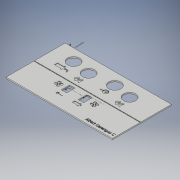
# Autodesk Inventor part: Caixa control - tapa
Saved by Autodesk Inventor 2019 (Build 230136000, 136)
## iProperties
Created: 2018-08-29
Part Number: Caixa control - tapa
Material: Genérico
Document SubType Name: Modeling
Designer: Albert Garangou Culebras
Density: 1 g/cm^3
Appearance: Valor por defecto
Author: Albert Garangou Culebras
Autodesk Inventor part; units mm, degrees
(part 1 of 2)
ref_plane "YZ Plane" through (0, 0, 0) normal (1, 0, 0) x (0, 1, 0)
ref_plane "XZ Plane" through (0, 0, 0) normal (0, 1, 0) x (-1, 0, 0)
ref_plane "XY Plane" through (0, 0, 0) normal (0, 0, 1) x (1, 0, 0)
sketch "Boceto1" plane through (0, 0, 0) normal (0, 1, 0) x (-1, 0, 0)
  line L0 (0, 0) -> (-180, 0)
  line L1 (-180, 0) -> (-180, -100)
  line L2 (-180, -100) -> (0, -100)
  line L3 (0, -100) -> (0, 0)
  dimension "d0" = 180
  dimension "d1" = 100
  constraints: 8 end point, 2 parallel, 1 horizontal, 1 perpendicular
  measures "d0" distance of L2.end L1.end
  measures "d1" distance of L1.end L0.end
extrude "base" add sketch "Boceto1" along normal blind 2
sketch "Boceto2" plane through (0, 2, 0) normal (0, 1, 0) x (1, 0, 0)
  line L0 (0, 100) -> (0, 0) projected
  line L1 (0, 0) -> (180, 0) projected
  line L2 (0, 100) -> (180, 100)
  line L3 (180, 100) -> (180, 0)
  line L4 (180, 0) -> (0, 0)
  line L5 (0, 0) -> (0, 100)
  line L6 (180, 50) -> (180, 0)
  line L7 (180, 0) -> (84.2308, 0)
  line L8 (180, 100) -> (0, 100) projected
  circle A0 centre (34.2888, 79.9235) radius 10.25
  circle A1 centre (104.2888, 79.9235) radius 10.25
  line L9 (65.4618, 35) -> (65.4618, 42)
  line L10 (65.4618, 42) -> (74.4618, 42)
  line L11 (74.4618, 42) -> (74.4618, 28)
  line L12 (74.4618, 28) -> (65.4618, 28)
  line L13 (65.4618, 28) -> (65.4618, 35)
  line L14 (94.2308, 35) -> (94.2308, 42)
  line L15 (103.2308, 42) -> (103.2308, 28)
  line L16 (103.2308, 28) -> (94.2308, 28)
  line L17 (94.2308, 28) -> (94.2308, 35)
  circle A2 centre (64.2888, 75.4263) radius 10.25
  circle A3 centre (134.2888, 74.9235) radius 10.25
  line L18 (94.2308, 42) -> (103.2308, 42)
  line L19 (94.2308, 42) -> (103.2308, 42)
  line L20 (94.2308, 42) -> (103.2308, 42)
  line L21 (103.2308, 42) -> (103.2308, 28)
  line L22 (103.2308, 28) -> (94.2308, 28)
  line L23 (94.2308, 28) -> (94.2308, 42)
  constraints: 42 end point, 8 perpendicular, 5 equal length, 4 centre point, 2 horizontal, 2 point on line, 2 vertical
sketch "Boceto5" plane through (0, 2, 0) normal (0, 1, 0) x (1, 0, 0)
  line L0 (37.6813, 63.0419) -> (37.6542, 60.4419) projected
  line L1 (37.6747, 62.4093) -> (37.6612, 61.1175)
  line L2 (41.6533, 62.4093) -> (37.6747, 62.4093)
  line L3 (41.6533, 62.4093) -> (44.1386, 62.4093) construction
  line L4 (44.1386, 62.4093) -> (44.1386, 58.5428) construction
  spline S0 degree 2 poles (41.6533, 62.4093) (44.1386, 62.4093) (44.1386, 58.5428) knots 1 1 1 2 2 2
  line L5 (41.6533, 61.1175) -> (42.896, 61.1175) construction
  line L6 (42.896, 61.1175) -> (42.896, 58.5428) construction
  spline S1 degree 2 poles (41.6533, 61.1175) (42.896, 61.1175) (42.896, 58.5428) knots 1 1 1 2 2 2
  line L7 (42.896, 58.5428) -> (44.1386, 58.5428)
  line L8 (37.6612, 61.1175) -> (41.6533, 61.1175)
  point P0 (0, 0)
  constraints: 8 end point, 3 horizontal, 2 point on line, 2 vertical, 6 other
extrude "Extrusión4" cut sketch "Boceto5" against normal blind 0.75
sketch "Boceto8" plane through (0, 2, 0) normal (0, 1, 0) x (1, 0, 0)
  spline S0 degree 4 poles (133.7635, 35.9708) (133.8407, 35.7147) (134.281, 35.6307) (134.3351, 35.9754) (134.306, 36.5115) (134.6867, 37.3994) (135.6799, 38.6611) (136.4874, 39.1799) (138.808, 38.5401) (139.0929, 36.16) knots 0 0 0 0 0 0.168165 0.246229 0.343173 0.454491 0.580711 1 1 1 1 1
  spline S1 degree 4 poles (139.0929, 36.16) (139.4262, 35.3106) (137.4111, 33.2429) (137.2359, 36.2151) (135.2011, 34.9657) knots 0 0 0 0 0 1 1 1 1 1
  spline S2 degree 3 poles (135.2011, 34.9657) (134.8312, 33.8706) (136.5984, 35.589) (138.0072, 32.8129) knots 0 0 0 0 1 1 1 1
  spline S3 degree 4 poles (134.6889, 32.599) (134.6741, 32.3205) (134.4844, 31.7908) (133.8798, 30.9164) (134.6566, 30.0496) (135.5938, 29.5497) (136.1798, 29.9491) (138.1553, 30.4347) (138.19, 32.1817) knots 0 0 0 0 0 0.26848 0.383335 0.491909 0.605906 1 1 1 1 1
  spline S4 degree 2 poles (138.19, 32.1817) (138.2278, 32.5571) (138.0072, 32.8129) knots 0 0 0 1 1 1
  spline S5 degree 3 poles (133.9221, 33.5854) (134.1222, 33.9496) (134.7297, 33.5872) (134.6889, 32.599) knots 0 0 0 0 1 1 1 1
  line L0 (134.19, 33.6433) -> (135.2195, 34.5853)
  line L1 (135.2195, 34.5853) -> (134.1584, 35.7449)
  spline S6 degree 2 poles (132.8663, 34.9339) (132.9078, 34.93) (132.9532, 34.9084) knots 0 0 0 1 1 1
  line L2 (132.9307, 34.9191) -> (132.9757, 34.8978) construction
  arc A0 (132.971, 34.8994) -> (132.935, 34.9165) centre (132.8007, 34.5869) ccw construction
  line L3 (132.9532, 34.4831) -> (134.1584, 35.7449)
  spline S7 degree 4 poles (133.9221, 33.5854) (133.6541, 32.8245) (133.8645, 27.8575) (126.9363, 31.5131) (129.6091, 34.4527) knots 0 0 0 0 0 1 1 1 1 1
  spline S8 degree 4 poles (131.5305, 34.2785) (131.5578, 34.2176) (132.6056, 34.0143) (133.4177, 34.5531) (132.9532, 34.9084) knots 0 0 0 0 0 1 1 1 1 1
  line L4 (133.0326, 34.5722) -> (133.9221, 33.5854)
  spline S9 degree 3 poles (129.6091, 34.4527) (129.986, 34.761) (130.8489, 34.796) (131.5305, 34.2785) knots 0 0 0 0 1 1 1 1
  spline S10 degree 3 poles (132.8663, 34.9339) (131.9784, 35.0507) (131.1917, 35.3523) (130.5912, 36.0652) knots 0 0 0 0 1 1 1 1
  spline S11 degree 3 poles (133.9221, 38.9749) (134.3989, 38.8274) (133.6923, 37.0279) (133.5207, 37.2609) knots 0 0 0 0 1 1 1 1
  spline S12 degree 2 poles (133.6277, 37.2803) (133.546, 36.3175) (133.7635, 35.9708) knots 0 0 0 1 1 1
  spline S13 degree 4 poles (130.5912, 36.0652) (130.1869, 36.2593) (129.7738, 37.4775) (130.529, 39.2025) (133.0958, 40.2641) (134.2584, 39.058) (134.0518, 38.316) knots 0 0 0 0 0 0.388226 0.566912 1 1 1 1 1
  spline S14 degree 4 poles (29.0799, 35.9708) (29.157, 35.7147) (29.5973, 35.6307) (29.6514, 35.9754) (29.6224, 36.5115) (30.003, 37.3994) (30.9963, 38.6611) (31.8038, 39.1799) (34.1243, 38.5401) (34.4092, 36.16) knots 0 0 0 0 0 0.168165 0.246229 0.343173 0.454491 0.580711 1 1 1 1 1
  spline S15 degree 4 poles (34.4092, 36.16) (34.7426, 35.3106) (32.7275, 33.2427) (32.5523, 36.2152) (30.5175, 34.9657) knots 0 0 0 0 0 1 1 1 1 1
  spline S16 degree 3 poles (30.5175, 34.9657) (30.1475, 33.8706) (31.9148, 35.589) (33.3235, 32.8129) knots 0 0 0 0 1 1 1 1
  spline S17 degree 4 poles (29.2384, 33.5854) (28.9711, 32.8226) (29.1762, 27.8661) (22.2595, 31.5004) (24.9254, 34.4527) knots 0 0 0 0 0 1 1 1 1 1
  spline S18 degree 3 poles (24.9254, 34.4527) (25.3024, 34.7608) (26.1651, 34.7964) (26.8468, 34.2785) knots 0 0 0 0 1 1 1 1
  spline S19 degree 3 poles (28.1827, 34.9339) (27.2948, 35.0506) (26.5081, 35.3522) (25.9075, 36.0652) knots 0 0 0 0 1 1 1 1
  spline S20 degree 3 poles (29.2384, 38.9749) (29.7153, 38.8274) (29.0086, 37.0279) (28.8371, 37.2609) knots 0 0 0 0 1 1 1 1
  spline S21 degree 2 poles (28.9441, 37.2803) (28.8529, 36.3252) (29.0799, 35.9708) knots 0 0 0 1 1 1
  spline S22 degree 4 poles (25.9075, 36.0652) (25.5031, 36.2596) (25.0894, 37.4781) (25.8441, 39.204) (28.412, 40.2654) (29.5744, 39.0581) (29.3681, 38.316) knots 0 0 0 0 0 0.388245 0.566915 1 1 1 1 1
  spline S23 degree 2 poles (28.1827, 34.9339) (28.2241, 34.93) (28.2695, 34.9084) knots 0 0 0 1 1 1
  line L5 (28.247, 34.9191) -> (28.2921, 34.8978) construction
  arc A1 (28.2873, 34.8994) -> (28.2513, 34.9165) centre (28.117, 34.5869) ccw construction
  spline S24 degree 4 poles (26.8468, 34.2785) (26.8742, 34.2176) (27.9219, 34.0143) (28.7341, 34.5531) (28.2695, 34.9084) knots 0 0 0 0 0 1 1 1 1 1
  line L6 (29.5064, 33.6433) -> (30.5358, 34.5853)
  line L7 (30.5358, 34.5853) -> (29.4747, 35.7449)
  line L8 (28.2695, 34.4831) -> (29.4747, 35.7449)
  line L9 (28.349, 34.5722) -> (29.2384, 33.5854)
  spline S25 degree 3 poles (29.2384, 33.5854) (29.458, 33.9209) (30.054, 33.5788) (30.0053, 32.599) knots 0 0 0 0 1 1 1 1
  spline S26 degree 4 poles (30.0053, 32.599) (29.9904, 32.3205) (29.8007, 31.7908) (29.1962, 30.9163) (29.973, 30.0496) (30.9102, 29.5497) (31.4961, 29.9491) (33.4717, 30.4347) (33.5063, 32.1817) knots 0 0 0 0 0 0.268482 0.383337 0.491912 0.605908 1 1 1 1 1
  spline S27 degree 2 poles (33.5063, 32.1817) (33.5446, 32.5566) (33.3235, 32.8129) knots 0 0 0 1 1 1
  spline S28 degree 4 poles (119.8733, 36.16) (120.2066, 35.3106) (118.1915, 33.2429) (118.0164, 36.2151) (115.9816, 34.9657) knots 0 0 0 0 0 1 1 1 1 1
  spline S29 degree 3 poles (115.9816, 34.9657) (115.6133, 33.8631) (117.371, 35.6191) (118.7876, 32.8129) knots 0 0 0 0 1 1 1 1
  spline S30 degree 4 poles (115.4694, 32.599) (115.4545, 32.3205) (115.2648, 31.7908) (114.6603, 30.9164) (115.4371, 30.0496) (116.3742, 29.5497) (116.9602, 29.9491) (118.9358, 30.4347) (118.9704, 32.1817) knots 0 0 0 0 0 0.26848 0.383334 0.491909 0.605906 1 1 1 1 1
  spline S31 degree 2 poles (118.9704, 32.1817) (119.0082, 32.5571) (118.7876, 32.8129) knots 0 0 0 1 1 1
  spline S32 degree 3 poles (114.7025, 33.5854) (114.9022, 33.9502) (115.5099, 33.5876) (115.4694, 32.599) knots 0 0 0 0 1 1 1 1
  line L10 (113.8233, 34.5828) -> (114.7025, 33.5854)
  line L11 (113.7111, 34.9191) -> (113.7562, 34.8978) construction
  arc A2 (113.7513, 34.8993) -> (113.7154, 34.9163) centre (113.6167, 34.6618) ccw construction
  spline S33 degree 2 poles (113.6467, 34.9339) (113.6939, 34.9273) (113.7336, 34.9084) knots 0 0 0 1 1 1
  spline S34 degree 4 poles (112.3109, 34.2785) (112.3408, 34.2198) (113.3726, 34.0011) (114.2222, 34.5748) (113.7336, 34.9084) knots 0 0 0 0 0 1 1 1 1 1
  spline S35 degree 4 poles (114.7025, 33.5854) (114.4345, 32.8245) (114.645, 27.8573) (107.7166, 31.5134) (110.3895, 34.4527) knots 0 0 0 0 0 1 1 1 1 1
  spline S36 degree 3 poles (110.3895, 34.4527) (110.7664, 34.761) (111.6293, 34.796) (112.3109, 34.2785) knots 0 0 0 0 1 1 1 1
  spline S37 degree 4 poles (114.5675, 35.9531) (114.7321, 35.7261) (115.0348, 35.6365) (115.1296, 35.9897) (115.0795, 36.5127) (115.4721, 37.4009) (116.453, 38.6597) (117.2768, 39.1811) (119.58, 38.5391) (119.8733, 36.16) knots 0 0 0 0 0 0.164455 0.241152 0.338745 0.450813 0.577884 1 1 1 1 1
  line L12 (114.9705, 33.6433) -> (115.9999, 34.5853)
  line L13 (115.9999, 34.5853) -> (114.9388, 35.7449)
  line L14 (113.7336, 34.4831) -> (114.9388, 35.7449)
  spline S38 degree 3 poles (113.6467, 34.9339) (112.7589, 35.0507) (111.9721, 35.3523) (111.3716, 36.0652) knots 0 0 0 0 1 1 1 1
  spline S39 degree 2 poles (114.4082, 37.2803) (114.3116, 36.3127) (114.5675, 35.9531) knots 0 0 0 1 1 1
  spline S40 degree 3 poles (114.7025, 38.9749) (115.1794, 38.8274) (114.4727, 37.0279) (114.3012, 37.2609) knots 0 0 0 0 1 1 1 1
  spline S41 degree 4 poles (111.3716, 36.0652) (110.9673, 36.2593) (110.5542, 37.4775) (111.3094, 39.2024) (113.8763, 40.2641) (115.0388, 39.058) (114.8322, 38.316) knots 0 0 0 0 0 0.388226 0.566912 1 1 1 1 1
  point P0 (0, 0)
  point P1 (134.0516, 35.7325)
  point P2 (134.2407, 35.8001)
  point P3 (134.3129, 36.0072)
  point P4 (134.34, 36.381)
  point P5 (134.6509, 37.2278)
  point P6 (135.2907, 38.1197)
  point P7 (135.9711, 38.6375)
  point P8 (137.147, 38.7049)
  point P9 (138.8595, 35.2829)
  point P10 (138.0532, 34.7967)
  point P11 (137.0489, 35.0292)
  point P12 (135.7604, 34.531)
  point P13 (134.5896, 32.1623)
  point P14 (134.3129, 31.4539)
  point P15 (134.2407, 30.7018)
  point P16 (134.7047, 30.0807)
  point P17 (135.2194, 29.809)
  point P18 (135.691, 29.7896)
  point P19 (136.7003, 30.1098)
  point P20 (138.1604, 32.5366)
  point P21 (133.6555, 32.4511)
  point P22 (134.4049, 33.5903)
  point P23 (134.1193, 33.7233)
  point P24 (132.4392, 30.9488)
  point P25 (132.3643, 34.2429)
  point P26 (130.0221, 31.3317)
  point P27 (131.623, 34.2428)
  point P28 (132.0101, 35.1224)
  point P29 (130.0107, 34.6379)
  point P30 (130.6834, 34.6496)
  point P31 (131.2628, 35.4731)
  point P32 (133.6396, 36.3337)
  point P33 (130.17, 36.6461)
  point P34 (133.6934, 39.3058)
  point P35 (130.1359, 37.7776)
  point P36 (132.3676, 39.6621)
  point P37 (130.8587, 38.9101)
  point P38 (29.3679, 35.7325)
  point P39 (29.5571, 35.8001)
  point P40 (29.6292, 36.0072)
  point P41 (29.6563, 36.381)
  point P42 (29.9672, 37.2278)
  point P43 (30.607, 38.1197)
  point P44 (31.2874, 38.6375)
  point P45 (32.4634, 38.7049)
  point P46 (34.1759, 35.2829)
  point P47 (33.3695, 34.7967)
  point P48 (32.3652, 35.0292)
  point P49 (31.0767, 34.531)
  point P50 (28.9716, 32.4513)
  point P51 (27.7553, 30.949)
  point P52 (25.3422, 31.3271)
  point P53 (25.3271, 34.6379)
  point P54 (25.9996, 34.6497)
  point P55 (27.3265, 35.1223)
  point P56 (26.5792, 35.473)
  point P57 (28.9506, 36.3421)
  point P58 (25.486, 36.6467)
  point P59 (25.4516, 37.7787)
  point P60 (26.1742, 38.9114)
  point P61 (27.6832, 39.6633)
  point P62 (29.0093, 39.3064)
  point P63 (26.9393, 34.2428)
  point P64 (27.6806, 34.2429)
  point P65 (29.4459, 33.7103)
  point P66 (29.7357, 33.5721)
  point P67 (29.9059, 32.1623)
  point P68 (29.6292, 31.4539)
  point P69 (29.557, 30.7018)
  point P70 (30.0211, 30.0807)
  point P71 (30.5358, 29.809)
  point P72 (31.0074, 29.7895)
  point P73 (32.0167, 30.1098)
  point P74 (33.477, 32.5361)
  point P75 (114.8834, 35.7384)
  point P76 (115.0212, 35.8001)
  point P77 (115.0933, 36.0072)
  point P78 (119.64, 35.2829)
  point P79 (118.8336, 34.7967)
  point P80 (117.8293, 35.0292)
  point P81 (116.5354, 34.538)
  point P82 (115.37, 32.1623)
  point P83 (115.0933, 31.4539)
  point P84 (115.0211, 30.7018)
  point P85 (115.4851, 30.0808)
  point P86 (115.9999, 29.809)
  point P87 (116.4714, 29.7896)
  point P88 (117.4807, 30.1098)
  point P89 (118.9408, 32.5366)
  point P90 (114.8994, 33.7235)
  point P91 (115.1849, 33.5908)
  point P92 (114.4359, 32.4511)
  point P93 (113.2196, 30.9488)
  point P94 (113.1447, 34.2429)
  point P95 (112.4034, 34.2428)
  point P96 (111.4638, 34.6496)
  point P97 (110.8024, 31.3318)
  point P98 (110.7911, 34.6379)
  point P99 (115.1204, 36.381)
  point P100 (115.4313, 37.2278)
  point P101 (116.0707, 38.1198)
  point P102 (116.7515, 38.6375)
  point P103 (117.9274, 38.7049)
  point P104 (112.7906, 35.1224)
  point P105 (112.0433, 35.4731)
  point P106 (114.42, 36.3337)
  point P107 (110.9504, 36.6461)
  point P108 (111.6392, 38.9101)
  point P109 (114.4738, 39.3058)
  point P110 (110.9164, 37.7776)
  point P111 (113.148, 39.6621)
  constraints: 30 end point, 6 midpoint, 3 centre point, 3 perpendicular, 3 point on circle, 219 other
sketch "Boceto6" plane through (0, 2, 0) normal (0, 1, 0) x (1, 0, 0)
  spline S0 degree 4 poles (54.0725, 35.9708) (54.1496, 35.7147) (54.59, 35.6307) (54.644, 35.9754) (54.615, 36.5115) (54.9956, 37.3994) (55.9889, 38.6611) (56.7964, 39.1799) (59.117, 38.5401) (59.4018, 36.16) knots 0 0 0 0 0 0.168165 0.246229 0.343173 0.454491 0.580711 1 1 1 1 1
  spline S1 degree 4 poles (59.4018, 36.16) (59.7352, 35.3106) (57.7201, 33.2427) (57.5449, 36.2152) (55.5101, 34.9657) knots 0 0 0 0 0 1 1 1 1 1
  spline S2 degree 3 poles (55.5101, 34.9657) (55.1402, 33.8706) (56.9074, 35.589) (58.3161, 32.8129) knots 0 0 0 0 1 1 1 1
  spline S3 degree 4 poles (54.2311, 33.5854) (53.9639, 32.8221) (54.1674, 27.8685) (47.254, 31.4971) (49.9181, 34.4527) knots 0 0 0 0 0 1 1 1 1 1
  spline S4 degree 3 poles (49.9181, 34.4527) (50.2951, 34.7607) (51.1577, 34.7965) (51.8394, 34.2785) knots 0 0 0 0 1 1 1 1
  spline S5 degree 3 poles (53.1753, 34.9339) (52.2874, 35.0506) (51.5007, 35.3522) (50.9002, 36.0652) knots 0 0 0 0 1 1 1 1
  spline S6 degree 3 poles (54.2311, 38.9749) (54.7079, 38.8274) (54.0012, 37.0279) (53.8297, 37.2609) knots 0 0 0 0 1 1 1 1
  spline S7 degree 2 poles (53.9367, 37.2803) (53.8441, 36.3262) (54.0725, 35.9708) knots 0 0 0 1 1 1
  spline S8 degree 4 poles (50.9002, 36.0652) (50.4957, 36.2597) (50.0819, 37.4782) (50.8365, 39.2042) (53.4046, 40.2656) (54.567, 39.0581) (54.3607, 38.316) knots 0 0 0 0 0 0.388247 0.566915 1 1 1 1 1
  spline S9 degree 2 poles (53.1753, 34.9339) (53.2167, 34.93) (53.2622, 34.9084) knots 0 0 0 1 1 1
  line L0 (53.2396, 34.9191) -> (53.2847, 34.8978) construction
  arc A0 (53.2799, 34.8994) -> (53.2439, 34.9165) centre (53.1096, 34.5869) ccw construction
  spline S10 degree 4 poles (51.8394, 34.2785) (51.8668, 34.2176) (52.9145, 34.0143) (53.7267, 34.5531) (53.2622, 34.9084) knots 0 0 0 0 0 1 1 1 1 1
  line L1 (54.499, 33.6433) -> (55.5284, 34.5853)
  line L2 (55.5284, 34.5853) -> (54.4673, 35.7449)
  line L3 (53.2622, 34.4831) -> (54.4673, 35.7449)
  line L4 (53.3416, 34.5722) -> (54.2311, 33.5854)
  spline S11 degree 3 poles (54.2311, 33.5854) (54.4552, 33.9139) (55.0489, 33.5768) (54.9979, 32.599) knots 0 0 0 0 1 1 1 1
  spline S12 degree 4 poles (54.9979, 32.599) (54.983, 32.3205) (54.7933, 31.7908) (54.1888, 30.9163) (54.9656, 30.0496) (55.9028, 29.5496) (56.4887, 29.9491) (58.4643, 30.4348) (58.4989, 32.1817) knots 0 0 0 0 0 0.268483 0.383338 0.491912 0.605909 1 1 1 1 1
  spline S13 degree 2 poles (58.4989, 32.1817) (58.5373, 32.5565) (58.3161, 32.8129) knots 0 0 0 1 1 1
  point P0 (0, 0)
  point P1 (54.3605, 35.7325)
  point P2 (54.5497, 35.8001)
  point P3 (54.6218, 36.0072)
  point P4 (54.649, 36.381)
  point P5 (54.9599, 37.2278)
  point P6 (55.5996, 38.1197)
  point P7 (56.28, 38.6375)
  point P8 (57.456, 38.7049)
  point P9 (59.1685, 35.2829)
  point P10 (58.3621, 34.7967)
  point P11 (57.3578, 35.0292)
  point P12 (56.0694, 34.531)
  point P13 (53.9642, 32.4514)
  point P14 (52.7478, 30.9491)
  point P15 (50.3358, 31.3259)
  point P16 (50.3197, 34.6378)
  point P17 (50.9922, 34.6497)
  point P18 (52.3191, 35.1223)
  point P19 (51.5719, 35.473)
  point P20 (53.9425, 36.3432)
  point P21 (50.4785, 36.6467)
  point P22 (50.4441, 37.7788)
  point P23 (51.1667, 38.9116)
  point P24 (52.6757, 39.6634)
  point P25 (54.0019, 39.3065)
  point P26 (51.9319, 34.2428)
  point P27 (52.6732, 34.2429)
  point P28 (54.4411, 33.7072)
  point P29 (54.7321, 33.5675)
  point P30 (54.8985, 32.1623)
  point P31 (54.6218, 31.4538)
  point P32 (54.5497, 30.7018)
  point P33 (55.0137, 30.0807)
  point P34 (55.5284, 29.8089)
  point P35 (56, 29.7895)
  point P36 (57.0093, 30.1098)
  point P37 (58.4697, 32.536)
  constraints: 10 end point, 2 midpoint, 1 centre point, 1 perpendicular, 1 point on circle, 73 other
sketch "Boceto10" plane through (0, 2, 0) normal (0, 1, 0) x (1, 0, 0)
  line L0 (128.9902, 8.9769) -> (181.2554, 8.9769) construction
  line L1 (181.2554, 8.9769) -> (181.2554, -0.3757) construction
  line L2 (181.2554, -0.3757) -> (128.9902, -0.3757) construction
  line L3 (128.9902, -0.3757) -> (128.9902, 8.9769) construction
  line L4 (128.9624, 4.4852) -> (130.4119, 8.7852)
  line L5 (130.4119, 8.7852) -> (131.1158, 8.7852)
  line L6 (131.1158, 8.7852) -> (132.5654, 4.4852)
  line L7 (132.5654, 4.4852) -> (131.9626, 4.4852)
  line L8 (131.9626, 4.4852) -> (131.5723, 5.6874)
  line L9 (131.5723, 5.6874) -> (129.9311, 5.6874)
  line L10 (129.9311, 5.6874) -> (129.5408, 4.4852)
  line L11 (129.5408, 4.4852) -> (128.9624, 4.4852)
  line L12 (131.4155, 6.1752) -> (130.75, 8.1998)
  line L13 (130.75, 8.1998) -> (130.0879, 6.1752)
  line L14 (130.0879, 6.1752) -> (131.4155, 6.1752)
  line L15 (133.4854, 4.4852) -> (132.9418, 4.4852)
  line L16 (132.9418, 4.4852) -> (132.9418, 8.9769)
  line L17 (132.9418, 8.9769) -> (133.4854, 8.9769)
  line L18 (133.4854, 8.9769) -> (133.4854, 4.4852)
  spline S0 degree 2 poles (136.9874, 6.1508) (136.9874, 5.3598) (136.2208, 4.3946) (135.6423, 4.3946) knots 0 0 0 1 2 2 2
  spline S1 degree 2 poles (135.6423, 4.3946) (135.381, 4.3946) (135.0081, 4.5235) (134.8269, 4.635) knots 0 0 0 1 2 2 2
  line L19 (134.8269, 4.635) -> (134.7921, 4.4852)
  line L20 (134.7921, 4.4852) -> (134.2833, 4.4852)
  line L21 (134.2833, 4.4852) -> (134.2833, 8.9769)
  line L22 (134.2833, 8.9769) -> (134.8269, 8.9769)
  line L23 (134.8269, 8.9769) -> (134.8269, 7.3739)
  spline S2 degree 2 poles (134.8269, 7.3739) (135.0325, 7.5586) (135.5099, 7.8025) (135.8131, 7.8025) knots 0 0 0 1 2 2 2
  spline S3 degree 2 poles (135.8131, 7.8025) (136.3602, 7.8025) (136.9874, 6.9279) (136.9874, 6.1508) knots 0 0 0 1 2 2 2
  spline S4 degree 2 poles (136.4264, 6.109) (136.4264, 6.6875) (136.0744, 7.2868) (135.6842, 7.2868) knots 0 0 0 1 2 2 2
  spline S5 degree 2 poles (135.6842, 7.2868) (135.4646, 7.2868) (135.0116, 7.0777) (134.8269, 6.9175) knots 0 0 0 1 2 2 2
  line L24 (134.8269, 6.9175) -> (134.8269, 5.0671)
  spline S6 degree 2 poles (134.8269, 5.0671) (135.0325, 4.9661) (135.3496, 4.8824) (135.5378, 4.8824) knots 0 0 0 1 2 2 2
  spline S7 degree 2 poles (135.5378, 4.8824) (135.9525, 4.8824) (136.4264, 5.4713) (136.4264, 6.109) knots 0 0 0 1 2 2 2
  spline S8 degree 2 poles (138.9527, 4.412) (138.1791, 4.412) (137.3289, 5.2797) (137.3289, 6.0812) knots 0 0 0 1 2 2 2
  spline S9 degree 2 poles (137.3289, 6.0812) (137.3289, 6.8687) (138.1547, 7.8025) (138.8203, 7.8025) knots 0 0 0 1 2 2 2
  spline S10 degree 2 poles (138.8203, 7.8025) (139.12, 7.8025) (139.5834, 7.6283) (139.7542, 7.4436) knots 0 0 0 1 2 2 2
  spline S11 degree 2 poles (139.7542, 7.4436) (139.9284, 7.2589) (140.1131, 6.7258) (140.1131, 6.339) knots 0 0 0 1 2 2 2
  line L25 (140.1131, 6.339) -> (140.1131, 6.0428)
  line L26 (140.1131, 6.0428) -> (137.8795, 6.0428)
  spline S12 degree 2 poles (137.8795, 6.0428) (137.8795, 5.4818) (138.444, 4.8859) (138.9457, 4.8859) knots 0 0 0 1 2 2 2
  spline S13 degree 2 poles (138.9457, 4.8859) (139.1235, 4.8859) (139.4684, 4.9661) (139.6078, 5.0288) knots 0 0 0 1 2 2 2
  spline S14 degree 2 poles (139.6078, 5.0288) (139.7542, 5.0985) (139.9563, 5.2205) (140.0225, 5.2762) knots 0 0 0 1 2 2 2
  line L27 (140.0225, 5.2762) -> (140.0538, 5.2762)
  line L28 (140.0538, 5.2762) -> (140.0538, 4.6838)
  spline S15 degree 2 poles (140.0538, 4.6838) (139.9598, 4.6455) (139.674, 4.534) (139.5625, 4.5026) knots 0 0 0 1 2 2 2
  spline S16 degree 2 poles (139.5625, 4.5026) (139.4057, 4.4573) (139.1478, 4.412) (138.9527, 4.412) knots 0 0 0 1 2 2 2
  spline S17 degree 2 poles (139.5834, 6.4575) (139.5765, 6.677) (139.4859, 6.9976) (139.3987, 7.1056) knots 0 0 0 1 2 2 2
  spline S18 degree 2 poles (139.3987, 7.1056) (139.3047, 7.2276) (139.0085, 7.3565) (138.7889, 7.3565) knots 0 0 0 1 2 2 2
  spline S19 degree 2 poles (138.7889, 7.3565) (138.5729, 7.3565) (138.2697, 7.2276) (138.1443, 7.1021) knots 0 0 0 1 2 2 2
  spline S20 degree 2 poles (138.1443, 7.1021) (138.0223, 6.9732) (137.8969, 6.6631) (137.8795, 6.4575) knots 0 0 0 1 2 2 2
  line L29 (137.8795, 6.4575) -> (139.5834, 6.4575)
  line L30 (142.3746, 7.13) -> (142.3467, 7.13)
  spline S21 degree 2 poles (142.3467, 7.13) (142.284, 7.1474) (142.1481, 7.1544) (142.054, 7.1544) knots 0 0 0 1 2 2 2
  spline S22 degree 2 poles (142.054, 7.1544) (141.8345, 7.1544) (141.4024, 6.9628) (141.2072, 6.7746) knots 0 0 0 1 2 2 2
  line L31 (141.2072, 6.7746) -> (141.2072, 4.4852)
  line L32 (141.2072, 4.4852) -> (140.6637, 4.4852)
  line L33 (140.6637, 4.4852) -> (140.6637, 7.7119)
  line L34 (140.6637, 7.7119) -> (141.2072, 7.7119)
  line L35 (141.2072, 7.7119) -> (141.2072, 7.2311)
  spline S23 degree 2 poles (141.2072, 7.2311) (141.5034, 7.4959) (141.946, 7.7119) (142.1551, 7.7119) knots 0 0 0 1 2 2 2
  spline S24 degree 2 poles (142.1551, 7.7119) (142.2387, 7.7119) (142.3223, 7.705) (142.3746, 7.6945) knots 0 0 0 1 2 2 2
  line L36 (142.3746, 7.6945) -> (142.3746, 7.13)
  spline S25 degree 2 poles (143.7719, 4.4225) (143.3294, 4.4225) (142.8311, 4.9277) (142.8311, 5.4748) knots 0 0 0 1 2 2 2
  line L37 (142.8311, 5.4748) -> (142.8311, 7.2624)
  line L38 (142.8311, 7.2624) -> (142.4652, 7.2624)
  line L39 (142.4652, 7.2624) -> (142.4652, 7.7119)
  line L40 (142.4652, 7.7119) -> (142.8311, 7.7119)
  line L41 (142.8311, 7.7119) -> (142.8311, 8.6389)
  line L42 (142.8311, 8.6389) -> (143.3747, 8.6389)
  line L43 (143.3747, 8.6389) -> (143.3747, 7.7119)
  line L44 (143.3747, 7.7119) -> (144.3748, 7.7119)
  line L45 (144.3748, 7.7119) -> (144.3748, 7.2624)
  line L46 (144.3748, 7.2624) -> (143.3747, 7.2624)
  line L47 (143.3747, 7.2624) -> (143.3747, 5.7257)
  spline S26 degree 2 poles (143.3747, 5.7257) (143.3747, 5.4818) (143.3921, 5.2135) (143.4513, 5.0985) knots 0 0 0 1 2 2 2
  spline S27 degree 2 poles (143.4513, 5.0985) (143.5001, 4.9974) (143.7196, 4.8964) (143.9078, 4.8964) knots 0 0 0 1 2 2 2
  spline S28 degree 2 poles (143.9078, 4.8964) (144.0402, 4.8964) (144.2876, 4.9765) (144.3434, 5.0009) knots 0 0 0 1 2 2 2
  line L48 (144.3434, 5.0009) -> (144.3748, 5.0009)
  line L49 (144.3748, 5.0009) -> (144.3748, 4.5131)
  spline S29 degree 2 poles (144.3748, 4.5131) (144.2214, 4.4713) (143.9078, 4.4225) (143.7719, 4.4225) knots 0 0 0 1 2 2 2
  spline S30 degree 2 poles (148.4657, 4.4016) (148.0092, 4.4016) (147.253, 4.6803) (146.9812, 4.9626) knots 0 0 0 1 2 2 2
  spline S31 degree 2 poles (146.9812, 4.9626) (146.7094, 5.2483) (146.4202, 6.0916) (146.4202, 6.6387) knots 0 0 0 1 2 2 2
  spline S32 degree 2 poles (146.4202, 6.6387) (146.4202, 7.1579) (146.7129, 7.9803) (146.9847, 8.273) knots 0 0 0 1 2 2 2
  spline S33 degree 2 poles (146.9847, 8.273) (147.2461, 8.5552) (148.0127, 8.8619) (148.4692, 8.8619) knots 0 0 0 1 2 2 2
  spline S34 degree 2 poles (148.4692, 8.8619) (148.6887, 8.8619) (149.0859, 8.7991) (149.2671, 8.7434) knots 0 0 0 1 2 2 2
  spline S35 degree 2 poles (149.2671, 8.7434) (149.4135, 8.7016) (149.7689, 8.5483) (149.8769, 8.4925) knots 0 0 0 1 2 2 2
  line L50 (149.8769, 8.4925) -> (149.8769, 7.8025)
  line L51 (149.8769, 7.8025) -> (149.8282, 7.8025)
  spline S36 degree 2 poles (149.8282, 7.8025) (149.7201, 7.8966) (149.4936, 8.0674) (149.2846, 8.1649) knots 0 0 0 1 2 2 2
  spline S37 degree 2 poles (149.2846, 8.1649) (149.1103, 8.2521) (148.6608, 8.3671) (148.403, 8.3671) knots 0 0 0 1 2 2 2
  spline S38 degree 2 poles (148.403, 8.3671) (147.7827, 8.3671) (147.0161, 7.4332) (147.0161, 6.6561) knots 0 0 0 1 2 2 2
  spline S39 degree 2 poles (147.0161, 6.6561) (147.0161, 6.224) (147.2182, 5.5759) (147.4098, 5.3529) knots 0 0 0 1 2 2 2
  spline S40 degree 2 poles (147.4098, 5.3529) (147.5945, 5.1299) (148.1172, 4.8964) (148.4448, 4.8964) knots 0 0 0 1 2 2 2
  spline S41 degree 2 poles (148.4448, 4.8964) (148.6852, 4.8964) (149.1661, 4.9661) (149.3299, 5.0358) knots 0 0 0 1 2 2 2
  line L52 (149.3299, 5.0358) -> (149.3299, 6.1474)
  line L53 (149.3299, 6.1474) -> (148.3333, 6.1474)
  line L54 (148.3333, 6.1474) -> (148.3333, 6.6491)
  line L55 (148.3333, 6.6491) -> (149.8944, 6.6491)
  line L56 (149.8944, 6.6491) -> (149.8944, 4.7709)
  spline S42 degree 2 poles (149.8944, 4.7709) (149.7863, 4.7222) (149.417, 4.5723) (149.2602, 4.527) knots 0 0 0 1 2 2 2
  spline S43 degree 2 poles (149.2602, 4.527) (149.0476, 4.4643) (148.7061, 4.4016) (148.4657, 4.4016) knots 0 0 0 1 2 2 2
  spline S44 degree 2 poles (152.3684, 4.8267) (152.3022, 4.7779) (152.0792, 4.6037) (151.9747, 4.5514) knots 0 0 0 1 2 2 2
  spline S45 degree 2 poles (151.9747, 4.5514) (151.8318, 4.4748) (151.5635, 4.3946) (151.3196, 4.3946) knots 0 0 0 1 2 2 2
  spline S46 degree 2 poles (151.3196, 4.3946) (151.1209, 4.3946) (150.762, 4.5444) (150.6261, 4.6803) knots 0 0 0 1 2 2 2
  spline S47 degree 2 poles (150.6261, 4.6803) (150.4972, 4.8128) (150.3404, 5.203) (150.3404, 5.4191) knots 0 0 0 1 2 2 2
  spline S48 degree 2 poles (150.3404, 5.4191) (150.3404, 5.7536) (150.6226, 6.2275) (150.9293, 6.3634) knots 0 0 0 1 2 2 2
  spline S49 degree 2 poles (150.9293, 6.3634) (151.2011, 6.4889) (151.9398, 6.5829) (152.3684, 6.6073) knots 0 0 0 1 2 2 2
  line L57 (152.3684, 6.6073) -> (152.3684, 6.7119)
  spline S50 degree 2 poles (152.3684, 6.7119) (152.3684, 6.9) (152.2534, 7.1335) (152.1489, 7.1997) knots 0 0 0 1 2 2 2
  spline S51 degree 2 poles (152.1489, 7.1997) (152.0444, 7.2659) (151.7447, 7.3077) (151.5844, 7.3077) knots 0 0 0 1 2 2 2
  spline S52 degree 2 poles (151.5844, 7.3077) (151.3962, 7.3077) (150.8875, 7.1962) (150.6331, 7.0882) knots 0 0 0 1 2 2 2
  line L58 (150.6331, 7.0882) -> (150.6017, 7.0882)
  line L59 (150.6017, 7.0882) -> (150.6017, 7.6423)
  spline S53 degree 2 poles (150.6017, 7.6423) (150.7516, 7.6841) (151.3126, 7.7886) (151.5879, 7.7886) knots 0 0 0 1 2 2 2
  spline S54 degree 2 poles (151.5879, 7.7886) (151.9224, 7.7886) (152.3789, 7.6841) (152.5601, 7.5482) knots 0 0 0 1 2 2 2
  spline S55 degree 2 poles (152.5601, 7.5482) (152.7378, 7.4158) (152.912, 6.9941) (152.912, 6.691) knots 0 0 0 1 2 2 2
  line L60 (152.912, 6.691) -> (152.912, 4.4852)
  line L61 (152.912, 4.4852) -> (152.3684, 4.4852)
  line L62 (152.3684, 4.4852) -> (152.3684, 4.8267)
  line L63 (152.3684, 5.2797) -> (152.3684, 6.1752)
  spline S56 degree 2 poles (152.3684, 6.1752) (152.1733, 6.1578) (151.5844, 6.0986) (151.3997, 6.0428) knots 0 0 0 1 2 2 2
  spline S57 degree 2 poles (151.3997, 6.0428) (151.1837, 5.9766) (150.9014, 5.7013) (150.9014, 5.4574) knots 0 0 0 1 2 2 2
  spline S58 degree 2 poles (150.9014, 5.4574) (150.9014, 5.1786) (151.215, 4.8964) (151.5147, 4.8964) knots 0 0 0 1 2 2 2
  spline S59 degree 2 poles (151.5147, 4.8964) (151.7691, 4.8964) (152.1872, 5.1159) (152.3684, 5.2797) knots 0 0 0 1 2 2 2
  line L64 (155.3861, 7.13) -> (155.3582, 7.13)
  spline S60 degree 2 poles (155.3582, 7.13) (155.2955, 7.1474) (155.1596, 7.1544) (155.0655, 7.1544) knots 0 0 0 1 2 2 2
  spline S61 degree 2 poles (155.0655, 7.1544) (154.846, 7.1544) (154.4139, 6.9628) (154.2188, 6.7746) knots 0 0 0 1 2 2 2
  line L65 (154.2188, 6.7746) -> (154.2188, 4.4852)
  line L66 (154.2188, 4.4852) -> (153.6752, 4.4852)
  line L67 (153.6752, 4.4852) -> (153.6752, 7.7119)
  line L68 (153.6752, 7.7119) -> (154.2188, 7.7119)
  line L69 (154.2188, 7.7119) -> (154.2188, 7.2311)
  spline S62 degree 2 poles (154.2188, 7.2311) (154.5149, 7.4959) (154.9575, 7.7119) (155.1666, 7.7119) knots 0 0 0 1 2 2 2
  spline S63 degree 2 poles (155.1666, 7.7119) (155.2502, 7.7119) (155.3338, 7.705) (155.3861, 7.6945) knots 0 0 0 1 2 2 2
  line L70 (155.3861, 7.6945) -> (155.3861, 7.13)
  spline S64 degree 2 poles (157.6058, 4.8267) (157.5396, 4.7779) (157.3166, 4.6037) (157.212, 4.5514) knots 0 0 0 1 2 2 2
  spline S65 degree 2 poles (157.212, 4.5514) (157.0692, 4.4748) (156.8008, 4.3946) (156.5569, 4.3946) knots 0 0 0 1 2 2 2
  spline S66 degree 2 poles (156.5569, 4.3946) (156.3583, 4.3946) (155.9994, 4.5444) (155.8635, 4.6803) knots 0 0 0 1 2 2 2
  spline S67 degree 2 poles (155.8635, 4.6803) (155.7346, 4.8128) (155.5778, 5.203) (155.5778, 5.4191) knots 0 0 0 1 2 2 2
  spline S68 degree 2 poles (155.5778, 5.4191) (155.5778, 5.7536) (155.86, 6.2275) (156.1666, 6.3634) knots 0 0 0 1 2 2 2
  spline S69 degree 2 poles (156.1666, 6.3634) (156.4384, 6.4889) (157.1772, 6.5829) (157.6058, 6.6073) knots 0 0 0 1 2 2 2
  line L71 (157.6058, 6.6073) -> (157.6058, 6.7119)
  spline S70 degree 2 poles (157.6058, 6.7119) (157.6058, 6.9) (157.4908, 7.1335) (157.3863, 7.1997) knots 0 0 0 1 2 2 2
  spline S71 degree 2 poles (157.3863, 7.1997) (157.2817, 7.2659) (156.982, 7.3077) (156.8218, 7.3077) knots 0 0 0 1 2 2 2
  spline S72 degree 2 poles (156.8218, 7.3077) (156.6336, 7.3077) (156.1248, 7.1962) (155.8705, 7.0882) knots 0 0 0 1 2 2 2
  line L72 (155.8705, 7.0882) -> (155.8391, 7.0882)
  line L73 (155.8391, 7.0882) -> (155.8391, 7.6423)
  spline S73 degree 2 poles (155.8391, 7.6423) (155.9889, 7.6841) (156.55, 7.7886) (156.8252, 7.7886) knots 0 0 0 1 2 2 2
  spline S74 degree 2 poles (156.8252, 7.7886) (157.1598, 7.7886) (157.6162, 7.6841) (157.7974, 7.5482) knots 0 0 0 1 2 2 2
  spline S75 degree 2 poles (157.7974, 7.5482) (157.9752, 7.4158) (158.1494, 6.9941) (158.1494, 6.691) knots 0 0 0 1 2 2 2
  line L74 (158.1494, 6.691) -> (158.1494, 4.4852)
  line L75 (158.1494, 4.4852) -> (157.6058, 4.4852)
  line L76 (157.6058, 4.4852) -> (157.6058, 4.8267)
  line L77 (157.6058, 5.2797) -> (157.6058, 6.1752)
  spline S76 degree 2 poles (157.6058, 6.1752) (157.4107, 6.1578) (156.8218, 6.0986) (156.6371, 6.0428) knots 0 0 0 1 2 2 2
  spline S77 degree 2 poles (156.6371, 6.0428) (156.421, 5.9766) (156.1388, 5.7013) (156.1388, 5.4574) knots 0 0 0 1 2 2 2
  spline S78 degree 2 poles (156.1388, 5.4574) (156.1388, 5.1786) (156.4524, 4.8964) (156.7521, 4.8964) knots 0 0 0 1 2 2 2
  spline S79 degree 2 poles (156.7521, 4.8964) (157.0064, 4.8964) (157.4246, 5.1159) (157.6058, 5.2797) knots 0 0 0 1 2 2 2
  line L78 (161.4458, 4.4852) -> (160.9022, 4.4852)
  line L79 (160.9022, 4.4852) -> (160.9022, 6.3251)
  spline S80 degree 2 poles (160.9022, 6.3251) (160.9022, 6.5481) (160.8604, 6.9314) (160.7977, 7.0464) knots 0 0 0 1 2 2 2
  spline S81 degree 2 poles (160.7977, 7.0464) (160.7315, 7.1683) (160.4945, 7.2868) (160.2924, 7.2868) knots 0 0 0 1 2 2 2
  spline S82 degree 2 poles (160.2924, 7.2868) (160.0903, 7.2868) (159.6617, 7.0708) (159.4561, 6.8966) knots 0 0 0 1 2 2 2
  line L80 (159.4561, 6.8966) -> (159.4561, 4.4852)
  line L81 (159.4561, 4.4852) -> (158.9125, 4.4852)
  line L82 (158.9125, 4.4852) -> (158.9125, 7.7119)
  line L83 (158.9125, 7.7119) -> (159.4561, 7.7119)
  line L84 (159.4561, 7.7119) -> (159.4561, 7.353)
  spline S83 degree 2 poles (159.4561, 7.353) (159.7, 7.5726) (160.1705, 7.8025) (160.4353, 7.8025) knots 0 0 0 1 2 2 2
  spline S84 degree 2 poles (160.4353, 7.8025) (160.9092, 7.8025) (161.4458, 7.1753) (161.4458, 6.5795) knots 0 0 0 1 2 2 2
  line L85 (161.4458, 6.5795) -> (161.4458, 4.4852)
  spline S85 degree 2 poles (162.3239, 3.9695) (162.3797, 3.9451) (162.5923, 3.8684) (162.7282, 3.8371) knots 0 0 0 1 2 2 2
  spline S86 degree 2 poles (162.7282, 3.8371) (162.878, 3.7987) (163.1324, 3.7534) (163.2822, 3.7534) knots 0 0 0 1 2 2 2
  spline S87 degree 2 poles (163.2822, 3.7534) (163.5331, 3.7534) (163.8816, 3.8859) (163.9791, 4.0043) knots 0 0 0 1 2 2 2
  spline S88 degree 2 poles (163.9791, 4.0043) (164.0732, 4.1228) (164.1464, 4.4329) (164.1464, 4.6316) knots 0 0 0 1 2 2 2
  line L86 (164.1464, 4.6316) -> (164.1464, 4.9138)
  spline S89 degree 2 poles (164.1464, 4.9138) (163.9269, 4.7222) (163.5052, 4.541) (163.1881, 4.541) knots 0 0 0 1 2 2 2
  spline S90 degree 2 poles (163.1881, 4.541) (162.6376, 4.541) (161.9859, 5.3598) (161.9859, 6.1299) knots 0 0 0 1 2 2 2
  spline S91 degree 2 poles (161.9859, 6.1299) (161.9859, 6.5307) (162.2124, 7.1509) (162.4006, 7.3705) knots 0 0 0 1 2 2 2
  spline S92 degree 2 poles (162.4006, 7.3705) (162.5818, 7.576) (163.0801, 7.8025) (163.3449, 7.8025) knots 0 0 0 1 2 2 2
  spline S93 degree 2 poles (163.3449, 7.8025) (163.5958, 7.8025) (163.9617, 7.6841) (164.1464, 7.576) knots 0 0 0 1 2 2 2
  line L87 (164.1464, 7.576) -> (164.1778, 7.7119)
  line L88 (164.1778, 7.7119) -> (164.69, 7.7119)
  line L89 (164.69, 7.7119) -> (164.69, 4.8546)
  spline S94 degree 2 poles (164.69, 4.8546) (164.69, 4.0322) (163.9756, 3.2656) (163.2404, 3.2656) knots 0 0 0 1 2 2 2
  spline S95 degree 2 poles (163.2404, 3.2656) (163.0034, 3.2656) (162.5086, 3.3423) (162.2961, 3.405) knots 0 0 0 1 2 2 2
  line L90 (162.2961, 3.405) -> (162.2961, 3.9695)
  line L91 (162.2961, 3.9695) -> (162.3239, 3.9695)
  line L92 (164.1464, 5.3598) -> (164.1464, 7.1335)
  spline S96 degree 2 poles (164.1464, 7.1335) (163.9443, 7.2311) (163.6028, 7.3147) (163.432, 7.3147) knots 0 0 0 1 2 2 2
  spline S97 degree 2 poles (163.432, 7.3147) (163.0209, 7.3147) (162.547, 6.7084) (162.547, 6.1404) knots 0 0 0 1 2 2 2
  spline S98 degree 2 poles (162.547, 6.1404) (162.547, 5.6038) (162.9059, 5.0427) (163.3101, 5.0427) knots 0 0 0 1 2 2 2
  spline S99 degree 2 poles (163.3101, 5.0427) (163.5226, 5.0427) (163.9687, 5.21) (164.1464, 5.3598) knots 0 0 0 1 2 2 2
  spline S100 degree 2 poles (168.1293, 6.0986) (168.1293, 5.2832) (167.3453, 4.3946) (166.6902, 4.3946) knots 0 0 0 1 2 2 2
  spline S101 degree 2 poles (166.6902, 4.3946) (166.0176, 4.3946) (165.2475, 5.3111) (165.2475, 6.0986) knots 0 0 0 1 2 2 2
  spline S102 degree 2 poles (165.2475, 6.0986) (165.2475, 6.907) (166.042, 7.8025) (166.6902, 7.8025) knots 0 0 0 1 2 2 2
  spline S103 degree 2 poles (166.6902, 7.8025) (167.3453, 7.8025) (168.1293, 6.9105) (168.1293, 6.0986) knots 0 0 0 1 2 2 2
  spline S104 degree 2 poles (167.5683, 6.0986) (167.5683, 6.7258) (167.1118, 7.3356) (166.6902, 7.3356) knots 0 0 0 1 2 2 2
  spline S105 degree 2 poles (166.6902, 7.3356) (166.2685, 7.3356) (165.8085, 6.7258) (165.8085, 6.0986) knots 0 0 0 1 2 2 2
  spline S106 degree 2 poles (165.8085, 6.0986) (165.8085, 5.4888) (166.2685, 4.8615) (166.6902, 4.8615) knots 0 0 0 1 2 2 2
  spline S107 degree 2 poles (166.6902, 4.8615) (167.1083, 4.8615) (167.5683, 5.4783) (167.5683, 6.0986) knots 0 0 0 1 2 2 2
  line L93 (171.1957, 4.4852) -> (170.6521, 4.4852)
  line L94 (170.6521, 4.4852) -> (170.6521, 4.8406)
  spline S108 degree 2 poles (170.6521, 4.8406) (170.4013, 4.6211) (169.9517, 4.3946) (169.673, 4.3946) knots 0 0 0 1 2 2 2
  spline S109 degree 2 poles (169.673, 4.3946) (169.4639, 4.3946) (169.091, 4.534) (168.9551, 4.6838) knots 0 0 0 1 2 2 2
  spline S110 degree 2 poles (168.9551, 4.6838) (168.8158, 4.8337) (168.6624, 5.2901) (168.6624, 5.6177) knots 0 0 0 1 2 2 2
  line L95 (168.6624, 5.6177) -> (168.6624, 7.7119)
  line L96 (168.6624, 7.7119) -> (169.206, 7.7119)
  line L97 (169.206, 7.7119) -> (169.206, 5.8721)
  spline S111 degree 2 poles (169.206, 5.8721) (169.206, 5.6142) (169.2444, 5.2762) (169.3106, 5.1508) knots 0 0 0 1 2 2 2
  spline S112 degree 2 poles (169.3106, 5.1508) (169.3768, 5.0253) (169.6033, 4.9103) (169.8158, 4.9103) knots 0 0 0 1 2 2 2
  spline S113 degree 2 poles (169.8158, 4.9103) (170.0145, 4.9103) (170.464, 5.1368) (170.6521, 5.3006) knots 0 0 0 1 2 2 2
  line L98 (170.6521, 5.3006) -> (170.6521, 7.7119)
  line L99 (170.6521, 7.7119) -> (171.1957, 7.7119)
  line L100 (171.1957, 7.7119) -> (171.1957, 4.4852)
  spline S114 degree 2 poles (175.5515, 4.4085) (175.1333, 4.4085) (174.426, 4.6908) (174.1681, 4.973) knots 0 0 0 1 2 2 2
  spline S115 degree 2 poles (174.1681, 4.973) (173.9102, 5.2518) (173.628, 6.0881) (173.628, 6.6317) knots 0 0 0 1 2 2 2
  spline S116 degree 2 poles (173.628, 6.6317) (173.628, 7.1718) (173.9033, 7.9733) (174.1646, 8.2695) knots 0 0 0 1 2 2 2
  spline S117 degree 2 poles (174.1646, 8.2695) (174.4225, 8.5587) (175.1264, 8.8619) (175.5619, 8.8619) knots 0 0 0 1 2 2 2
  spline S118 degree 2 poles (175.5619, 8.8619) (175.778, 8.8619) (176.1578, 8.7991) (176.3181, 8.7504) knots 0 0 0 1 2 2 2
  spline S119 degree 2 poles (176.3181, 8.7504) (176.4575, 8.7051) (176.7467, 8.5761) (176.8896, 8.4995) knots 0 0 0 1 2 2 2
  line L101 (176.8896, 8.4995) -> (176.8896, 7.8095)
  line L102 (176.8896, 7.8095) -> (176.8443, 7.8095)
  spline S120 degree 2 poles (176.8443, 7.8095) (176.7676, 7.8792) (176.5307, 8.0743) (176.3599, 8.1684) knots 0 0 0 1 2 2 2
  spline S121 degree 2 poles (176.3599, 8.1684) (176.1961, 8.259) (175.8094, 8.374) (175.5585, 8.374) knots 0 0 0 1 2 2 2
  spline S122 degree 2 poles (175.5585, 8.374) (175.2832, 8.374) (174.7919, 8.1475) (174.6072, 7.9315) knots 0 0 0 1 2 2 2
  spline S123 degree 2 poles (174.6072, 7.9315) (174.426, 7.7119) (174.2239, 7.0464) (174.2239, 6.6317) knots 0 0 0 1 2 2 2
  spline S124 degree 2 poles (174.2239, 6.6317) (174.2239, 6.1892) (174.4364, 5.5515) (174.6211, 5.332) knots 0 0 0 1 2 2 2
  spline S125 degree 2 poles (174.6211, 5.332) (174.8023, 5.1194) (175.2867, 4.9034) (175.5585, 4.9034) knots 0 0 0 1 2 2 2
  spline S126 degree 2 poles (175.5585, 4.9034) (175.8059, 4.9034) (176.2275, 5.0253) (176.3913, 5.1159) knots 0 0 0 1 2 2 2
  spline S127 degree 2 poles (176.3913, 5.1159) (176.5481, 5.2065) (176.7816, 5.3947) (176.8478, 5.4609) knots 0 0 0 1 2 2 2
  line L103 (176.8478, 5.4609) -> (176.8896, 5.4609)
  line L104 (176.8896, 5.4609) -> (176.8896, 4.7779)
  spline S128 degree 2 poles (176.8896, 4.7779) (176.7467, 4.7117) (176.4958, 4.5897) (176.3181, 4.534) knots 0 0 0 1 2 2 2
  spline S129 degree 2 poles (176.3181, 4.534) (176.1299, 4.4713) (175.8094, 4.4085) (175.5515, 4.4085) knots 0 0 0 1 2 2 2
  point P0 (0, 0)
  constraints: 2 other
extrude "Extrusión8" cut sketch "Boceto10" against normal blind 0.5
sketch "Boceto11" plane through (0, 0, 0) normal (0, -1, 0) x (1, 0, 0)
  line L0 (10.005, -7.4262) -> (-19.8869, -7.4262) construction
  line L1 (-19.8869, -7.4262) -> (-19.8869, 2.4029) construction
  line L2 (-19.8869, 2.4029) -> (10.005, 2.4029) construction
  line L3 (10.005, 2.4029) -> (10.005, -7.4262) construction
  line L4 (7.6083, -4.8816) -> (7.9406, -4.8816)
  line L5 (7.9406, -4.8816) -> (7.9406, -7.0351)
  line L6 (7.9406, -7.0351) -> (8.5929, -5.5704)
  line L7 (8.5929, -5.5704) -> (8.7955, -5.5704)
  line L8 (8.7955, -5.5704) -> (9.4418, -7.0351)
  line L9 (9.4418, -7.0351) -> (9.4418, -4.8816)
  line L10 (9.4418, -4.8816) -> (9.7518, -4.8816)
  line L11 (9.7518, -4.8816) -> (9.7518, -7.3816)
  line L12 (9.7518, -7.3816) -> (9.298, -7.3816)
  line L13 (9.298, -7.3816) -> (8.674, -5.9898)
  line L14 (8.674, -5.9898) -> (8.0703, -7.3816)
  line L15 (8.0703, -7.3816) -> (7.6083, -7.3816)
  line L16 (7.6083, -7.3816) -> (7.6083, -4.8816)
  line L17 (6.5184, -4.8816) -> (6.5184, -7.0858)
  line L18 (6.5184, -7.0858) -> (7.3571, -7.0858)
  line L19 (7.3571, -7.0858) -> (7.3571, -7.3816)
  line L20 (7.3571, -7.3816) -> (5.3474, -7.3816)
  line L21 (5.3474, -7.3816) -> (5.3474, -7.0858)
  line L22 (5.3474, -7.0858) -> (6.1861, -7.0858)
  line L23 (6.1861, -7.0858) -> (6.1861, -4.8816)
  line L24 (6.1861, -4.8816) -> (6.5184, -4.8816)
  spline S0 degree 2 poles (4.1177, -4.837) (4.3608, -4.837) (4.772, -5.0011) (4.922, -5.1652) knots 0 0 0 1 2 2 2
  spline S1 degree 2 poles (4.922, -5.1652) (5.0719, -5.3273) (5.236, -5.8135) (5.236, -6.1296) knots 0 0 0 1 2 2 2
  spline S2 degree 2 poles (5.236, -6.1296) (5.236, -6.4436) (5.0759, -6.9095) (4.924, -7.0817) knots 0 0 0 1 2 2 2
  spline S3 degree 2 poles (4.924, -7.0817) (4.7741, -7.2499) (4.3648, -7.4262) (4.1116, -7.4262) knots 0 0 0 1 2 2 2
  spline S4 degree 2 poles (4.1116, -7.4262) (3.986, -7.4262) (3.7652, -7.3897) (3.672, -7.3613) knots 0 0 0 1 2 2 2
  spline S5 degree 2 poles (3.672, -7.3613) (3.5909, -7.335) (3.4228, -7.26) (3.3397, -7.2155) knots 0 0 0 1 2 2 2
  line L25 (3.3397, -7.2155) -> (3.3397, -6.8143)
  line L26 (3.3397, -6.8143) -> (3.366, -6.8143)
  spline S6 degree 2 poles (3.366, -6.8143) (3.4106, -6.8548) (3.5484, -6.9683) (3.6476, -7.023) knots 0 0 0 1 2 2 2
  spline S7 degree 2 poles (3.6476, -7.023) (3.7429, -7.0757) (3.9677, -7.1425) (4.1136, -7.1425) knots 0 0 0 1 2 2 2
  spline S8 degree 2 poles (4.1136, -7.1425) (4.2737, -7.1425) (4.5593, -7.0108) (4.6667, -6.8852) knots 0 0 0 1 2 2 2
  spline S9 degree 2 poles (4.6667, -6.8852) (4.772, -6.7576) (4.8895, -6.3706) (4.8895, -6.1296) knots 0 0 0 1 2 2 2
  spline S10 degree 2 poles (4.8895, -6.1296) (4.8895, -5.8723) (4.766, -5.5015) (4.6586, -5.3739) knots 0 0 0 1 2 2 2
  spline S11 degree 2 poles (4.6586, -5.3739) (4.5532, -5.2503) (4.2716, -5.1247) (4.1136, -5.1247) knots 0 0 0 1 2 2 2
  spline S12 degree 2 poles (4.1136, -5.1247) (3.9698, -5.1247) (3.7246, -5.1956) (3.6294, -5.2483) knots 0 0 0 1 2 2 2
  spline S13 degree 2 poles (3.6294, -5.2483) (3.5382, -5.3009) (3.4025, -5.4103) (3.364, -5.4488) knots 0 0 0 1 2 2 2
  line L27 (3.364, -5.4488) -> (3.3397, -5.4488)
  line L28 (3.3397, -5.4488) -> (3.3397, -5.0518)
  spline S14 degree 2 poles (3.3397, -5.0518) (3.4228, -5.0133) (3.5686, -4.9424) (3.672, -4.9099) knots 0 0 0 1 2 2 2
  spline S15 degree 2 poles (3.672, -4.9099) (3.7814, -4.8735) (3.9677, -4.837) (4.1177, -4.837) knots 0 0 0 1 2 2 2
  point P0 (0, 0)
  constraints: 2 other
extrude "Extrusión9" cut sketch "Boceto11" against normal blind 0.3
sketch "Boceto12" plane through (0, 2, 0) normal (0, 1, 0) x (1, 0, 0)
  line L0 (89.4618, 42) -> (98.4618, 42) projected
  line L1 (0, 47.5) -> (0, 48)
  line L2 (0, 100) -> (0, 0) projected
  line L3 (0, 47.5) -> (0, 47)
  line L4 (0, 47) -> (180, 47)
  line L5 (0, 48) -> (180, 48)
  line L6 (180, 47) -> (180, 48)
  constraints: 10 end point, 2 point on line
extrude "Extrusión11" cut sketch "Boceto12" against normal blind 0.3